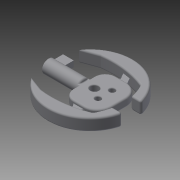
# Autodesk Inventor part: Concealed Cuff Key
Saved by Autodesk Inventor 2014 (Build 180170000, 170)
## iProperties
Created: 2014-03-28
Part Number: Concealed Cuff Key
Material: Generic
Document SubType Name: Modeling
Designer: s601298
Density: 1 g/cm^3
Appearance: Default
Author: s601298
Autodesk Inventor part; units mm, degrees
ref_plane "YZ Plane" through (0, 0, 0) normal (1, 0, 0) x (0, 1, 0)
ref_plane "XZ Plane" through (0, 0, 0) normal (0, 1, 0) x (-1, 0, 0)
sketch "Sketch1" plane through (0, 0, 0) normal (1, 0, 0) x (0, 1, 0)
  arc A0 (0.825, -1.6279) -> (-0.825, -1.6279) centre (0, 0) ccw
  circle A1 centre (0, 0) radius 1.15
  line L0 (-0.825, -1.6279) -> (-0.825, -4.0999)
  line L1 (0.825, -1.6279) -> (0.825, -4.0999)
  line L2 (-0.825, -4.0999) -> (0.825, -4.0999)
  dimension "d2" = 2.472
  dimension "d3" = 2.472
  dimension "d4" = 1.65
  constraints: 6 end point, 2 centre point, 2 coincident, 2 point on circle, 1 parallel, 1 perpendicular, 1 vertical
  measures "d2" distance of L0.start L0.end
  measures "d3" distance of L1.start L1.end
  measures "d4" distance of L0.end L1.end
extrude "Extrusion1" add sketch "Sketch1" along normal blind 3
sketch "Sketch2" plane through (3, 0, 0) normal (1, 0, 0) x (0, 0, -1)
  circle A0 centre (0, 0) radius 1.15 projected
  arc A1 (1.6279, 0.825) -> (1.6279, -0.825) centre (0, 0) ccw projected
  circle A2 centre (0, 0) radius 1.15
  circle A3 centre (0, 0) radius 1.825
  constraints: 2 centre point, 2 coincident, 2 concentric
extrude "Extrusion2" add sketch "Sketch2" along normal blind 2
sketch "Sketch3" plane through (5, 0, 0) normal (1, 0, 0) x (0, 0, -1)
  circle A0 centre (0, 0) radius 1.825 projected
  circle A1 centre (0, 0) radius 1.825
  constraints: 1 centre point, 1 coincident, 1 concentric
extrude "Extrusion3" add sketch "Sketch3" along normal blind 5
sketch "Sketch4" plane through (10, 0, 0) normal (1, 0, 0) x (0, 0, -1)
  circle A0 centre (0, 0) radius 1.825 projected
  line L0 (-6, 1.15) -> (6, 1.15)
  line L1 (6, 1.15) -> (6, -1.15)
  line L2 (6, -1.15) -> (-6, -1.15)
  line L3 (-6, -1.15) -> (-6, 1.15)
  dimension "d12" = 12
  dimension "d13" = 1.15
  dimension "d14" = 1.15
  dimension "d15" = 6
  constraints: 8 end point, 2 parallel, 1 horizontal, 1 perpendicular
  measures "d12" distance of L0.start L0.end
  measures "d13" distance from line of A0.centre L0
  measures "d14" distance from line of L2 A0.centre
  measures "d15" distance from line of A0.centre L3
extrude "Extrusion4" add sketch "Sketch4" along normal blind 10 contours A0 L2 L0 | A0 L0 L1 L2 | A0 L2 L3 L0
fillet "Fillet1" radius 4 2 edges at (20, 0, -6) (20, 0, 6)
fillet "Fillet2" radius 3 2 edges at (10, 0, -6) (10, 0, 6)
fillet "Fillet4" radius 0.5 10 edges at (10, -1.15, -2.2085) (14.5, -1.15, -6) (18.8284, -1.15, -4.8284) (20, -1.15, 0) (18.8284, -1.15, 4.8284) (14.5, -1.15, 6) (10.8787, -1.15, 5.1213) (10, -1.15, 2.2085) (10.8787, -1.15, -5.1213) (10, -1.825, 0)
fillet "Fillet5" radius 0.5 10 edges at (10, 1.825, 0) (10, 1.15, 2.2085) (14.5, 1.15, 6) (18.8284, 1.15, 4.8284) (20, 1.15, 0) (18.8284, 1.15, -4.8284) (14.5, 1.15, -6) (10.8787, 1.15, -5.1213) (10, 1.15, -2.2085) (10.8787, 1.15, 5.1213)
fillet "Fillet6" radius 0.25 4 edges at (10, 1.15, 1.4171) (10, 1.15, -1.4171) (10, -1.15, 1.4171) (10, -1.15, -1.4171)
fillet "Fillet7" radius 0.25 10 edges at (9.9526, -1.15, 1.0206) (9.6538, -1.1211, 1.4092) (9.9526, -1.15, -1.0206) (9.6538, -1.1211, -1.4092) (10, -1.15, 0) (9.9526, 1.15, -1.0206) (9.6538, 1.1211, -1.4092) (9.9526, 1.15, 1.0206) (9.6538, 1.1211, 1.4092) (10, 1.15, 0)
sketch "Sketch7" plane through (13, -1.15, -5.5) normal (0, -1, 0) x (1, 0, 0)
  arc A0 (3, 0) -> (6.5, 3.5) centre (3, 3.5) ccw projected
  arc A1 (6.5, 7.5) -> (3, 11) centre (3, 7.5) ccw projected
  circle A2 centre (3, 7.5) radius 0.75
  circle A3 centre (3, 3.5) radius 0.75
  circle A4 centre (0, 5.5) radius 1.125
  point P0 (-13, 5.5)
  dimension "d27" = 1.5
  dimension "d28" = 1.5
  dimension "d29" = 2.25
  constraints: 3 centre point, 2 coincident
  measures "d27" diameter of A2
  measures "d28" diameter of A3
  measures "d29" diameter of A4
extrude "Extrusion5" cut sketch "Sketch7" against normal blind 8
fillet "Fillet8" radius 0.25 6 edges at (15.25, -1.15, 2) (11.875, -1.15, 0) (11.875, 1.15, 0) (15.25, 1.15, 2) (15.25, 1.15, -2) (15.25, -1.15, -2)
ref_plane "Work Plane1" through (13, 0, -5.5) normal (0, -1, 0) x (1, 0, 0)
sketch "Sketch9" plane through (13, 0, -5.5) normal (0, -1, 0) x (1, 0, 0)
  arc A0 (-11.1323, -1.1977) -> (-11.1323, 12.1977) centre (-1.1754, 5.5) ccw
  line L0 (-11.1323, 12.1977) -> (-6.607, 13.8449)
  arc A1 (6.1921, -1.1977) -> (6.1921, 12.1977) centre (-6.1018, 5.5) ccw
  arc A2 (6.1921, 12.1977) -> (-6.607, 13.8449) centre (-3.3884, -11.6957) ccw
  line L1 (-13, 5.5) -> (12.9218, 5.5)
  line L2 (-11.1323, -1.1977) -> (-6.607, -2.8449)
  arc A3 (-6.607, -2.8449) -> (6.1921, -1.1977) centre (-3.3884, 22.6957) ccw
  dimension "d33" = 24
  dimension "d34" = 14
  constraints: 8 point on circle, 6 end point, 4 centre point, 2 symmetric about line, 1 horizontal, 1 other
  measures "d33" diameter of A0
  measures "d34" radius of A1
extrude "Extrusion6" add sketch "Sketch9" along normal mid plane 3.5
sketch "Sketch10" plane through (13, 0, -5.5) normal (0, -1, 0) x (1, 0, 0)
  line L0 (-13, 5.5) -> (12.0692, 5.5)
  line L1 (3, 11.5) -> (0, 11.5) projected
  arc A0 (7, 7.5) -> (3, 11.5) centre (3, 7.5) ccw projected
  line L2 (7, 3.5) -> (7, 7.5) projected
  arc A1 (3, -0.5) -> (7, 3.5) centre (3, 3.5) ccw projected
  line L3 (0, -0.5) -> (3, -0.5) projected
  arc A2 (6.1921, 12.1977) -> (-6.607, 13.8449) centre (-3.3884, -11.6957) ccw projected
  arc A3 (6.1921, -1.1977) -> (6.1921, 12.1977) centre (-6.1018, 5.5) ccw projected
  arc A4 (-6.607, -2.8449) -> (6.1921, -1.1977) centre (-3.3884, 22.6957) ccw projected
  line L4 (0, -0.5) -> (0.6428, -1.266)
  line L5 (0, -0.5) -> (1, -0.5) construction
  line L6 (0.6428, -1.266) -> (-0.2764, -2.8581)
  line L7 (0, 11.5) -> (0.6428, 12.266)
  line L8 (0, 11.5) -> (1, 11.5) construction
  line L9 (0.6428, 12.266) -> (-0.2764, 13.8581)
  line L10 (3, 11.5) -> (1.8392, 13.5106)
  line L11 (3, 11.5) -> (5.3216, 11.5) construction
  line L12 (3, -0.5) -> (1.8392, -2.5106)
  line L13 (3, -0.5) -> (5.3216, -0.5) construction
  dimension "d37" = 1
  dimension "d38" = 50
  dimension "d39" = 110
  dimension "d40" = 1
  dimension "d41" = 50
  dimension "d42" = 110
  dimension "d43" = 120
  dimension "d44" = 120
  constraints: 22 end point, 5 horizontal, 4 equal length, 4 point on circle
  measures "d37" distance of L3.start L4.end
  measures "d38" angle of L4 L5
  measures "d39" angle of L4 L6
  measures "d40" distance of L1.end L7.end
  measures "d41" angle of L8 L7
  measures "d42" angle of L9 L7
  measures "d43" angle of L11 L10
  measures "d44" angle of L12 L13
extrude "Extrusion7" add sketch "Sketch10" along normal mid plane 0.8 contours L12 A4 L6 L4 L3 | L1 L7 L9 A2 L10
sketch "Sketch11" plane through (13, 1.75, -5.5) normal (0, 1, 0) x (1, 0, 0)
  arc A0 (-11.1323, -12.1977) -> (-11.1323, 1.1977) centre (-1.1754, -5.5) ccw projected
  arc A1 (6.1921, -12.1977) -> (6.1921, 1.1977) centre (-6.1018, -5.5) ccw projected
  line L0 (7.6473, -2.8617) -> (10.531, -2.8617)
  line L1 (7.6473, -8.1383) -> (10.531, -8.1383)
  point P0 (-13, -5.5)
  constraints: 4 end point, 4 point on circle, 1 parallel
extrude "Extrusion8" cut sketch "Sketch11" against normal blind 10
fillet "Fillet9" radius 0.5 14 edges at (12.8974, 1.75, -8.3364) (12.8974, -1.75, -8.3364) (6.393, 0, -8.3449) (4.1303, 1.75, -7.5213) (4.1303, -1.75, -7.5213) (14.0348, 1.75, -11.7947) (22.0892, 1.75, -2.6383) (22.0892, -1.75, -2.6383) (20.6473, 0, -2.6383) (20.077, -1.75, -4.7244) (20.077, 1.75, -4.7244) (19.1921, 0, -6.6977) (23.531, 0, -2.6383) (14.0348, -1.75, -11.7947)
fillet "Fillet10" radius 0.5 14 edges at (22.0892, 1.75, 2.6383) (22.0892, -1.75, 2.6383) (20.6473, 0, 2.6383) (23.531, 0, 2.6383) (14.0348, -1.75, 11.7947) (20.077, -1.75, 4.7244) (20.077, 1.75, 4.7244) (19.1921, 0, 6.6977) (12.8974, -1.75, 8.3364) (12.8974, 1.75, 8.3364) (4.1303, -1.75, 7.5213) (6.393, 0, 8.3449) (4.1303, 1.75, 7.5213) (14.0348, 1.75, 11.7947)
body "Solid1"
